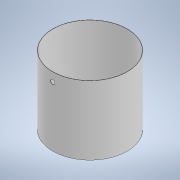
# Autodesk Inventor part: fish tank 1
Saved by Autodesk Inventor 2020 (Build 240168000, 168)
## iProperties
Created: 2019-09-26
Part Number: fish tank 1
Material: Generic
Document SubType Name: Modeling
Designer: Abbas
Density: 1 g/cm^3
Appearance: Default
Author: Abbas
Autodesk Inventor part; units mm, degrees
ref_plane "YZ Plane" through (0, 0, 0) normal (1, 0, 0) x (0, 1, 0)
ref_plane "XZ Plane" through (0, 0, 0) normal (0, 1, 0) x (-1, 0, 0)
sketch "Sketch1" plane through (0, 0, 0) normal (0, 1, 0) x (-1, 0, 0)
  circle A0 centre (0, 0) radius 1275
  dimension "d0" = 2550
  constraints: 1 centre point, 1 coincident
  measures "d0" diameter of A0
extrude "Extrusion1" add sketch "Sketch1" along normal blind 2350
sketch "Sketch2" plane through (0, 2350, 0) normal (0, 1, 0) x (1, 0, 0)
  circle A0 centre (0, 0) radius 1265
  dimension "d3" = 2530
  constraints: 1 centre point, 1 coincident
  measures "d3" diameter of A0
extrude "Extrusion2" cut sketch "Sketch2" against normal blind 2330
ref_plane "Work Plane2" through (0, 0, 1275) normal (0, 0, 1) x (1, 0, 0)
sketch "Sketch3" plane through (0, 0, 1275) normal (0, 0, 1) x (1, 0, 0)
  circle A0 centre (0, 2050) radius 75
  line L0 (1275, 2350) -> (-1275, 2350) projected
  point P0 (0, 0)
  dimension "d6" = 150
  dimension "d7" = 300
  constraints: 1 centre point
  measures "d6" diameter of A0
  measures "d7" distance from line of A0.centre L0
extrude "Extrusion3" cut sketch "Sketch3" against normal blind 30
body "Solid1"
